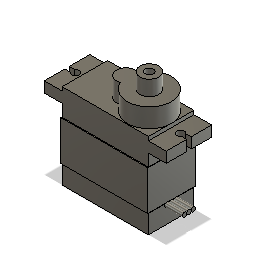
MG90_Rebuild (Autodesk Fusion 360 design; units mm, degrees)
Autodesk Fusion 360 part; units mm, degrees
note: some values were not read from the file. Set by a fixed rule: which sketch regions a step uses.
sketch "ServoRotatingPlate" plane through (0, 0, 0) normal (0, 1, 0) x (1, 0, 0)
  circle A0 centre (0, 0) radius 5.8
  line L0 (5.75, 6) -> (-17.05, 6)
  line L1 (-17.05, 6) -> (-17.05, -6)
  line L2 (-17.05, -6) -> (5.75, -6)
  line L3 (5.75, -6) -> (5.75, 6)
  line L4 (-8.7, 0) -> (5.75, 0) construction
  circle A1 centre (-6.2, 0) radius 2.5
  circle A2 centre (0, 0) radius 2.5
  circle A3 centre (0, 0) radius 1.1
  point P0 (5.8, 0)
  dimension "d4" = 11.6
  dimension "d6" = 12
  dimension "d7" = 22.8
  dimension "d10" = 5
  dimension "d12" = 14.5
  dimension "d13" = 5.75
  dimension "d14" = 8.1
  dimension "d48" = 5
  dimension "d49" = 1.4
  constraint coincident A0.centre A2.centre
  constraint horizontal L0
  constraint vertical L1
  constraint horizontal L2
  constraint vertical L3
  constraint horizontal L4
  constraint midpoint L3 L4.end
  constraint coincident L4 A1.centre
  constraint coincident L4.start A1
  constraint coincident A0.centre L4
  constraint coincident L4 P0
  constraint coincident A0 P0
  constraint concentric A0 A2
  constraint concentric A2 A3
  measures "d4" diameter of A0
  measures "d6" distance of L0.start L2.end
  measures "d7" distance of L0.start L0.end
  measures "d10" diameter of A1
  measures "d12" distance of L4.start P0
  measures "d13" distance of A0.centre L3
  measures "d48" diameter of A2
  measures "d49" distance of A2 A3
extrude "Extrude1" add sketch "ServoRotatingPlate" against normal blind 5 contours A0 L3 | A0 L3 A1 | A0 A1 | A0 A1 | A2 | A3
extrude "Extrude2" add sketch "ServoRotatingPlate" against normal blind 22.5 from surface at -5 contours A0 L3 A1 | A0 L0 L1 L2 L3 A1 | A0 A1 | A0 A1 | A2 | A3
ref_plane "WorkPlane1" through (-5.65, -6, 0) normal (0, 1, 0) x (0, 0, 1)
sketch "EarBase" plane through (-5.65, -6, 0) normal (0, 1, 0) x (1, 0, 0)
  line L0 (16.1, 6) -> (-16.1, 6)
  line L1 (-16.1, 6) -> (-16.1, -6)
  line L2 (-16.1, -6) -> (16.1, -6)
  line L3 (16.1, -6) -> (16.1, 6)
  line L4 (16.1, 6) -> (-16.1, -6) construction
  line L5 (-16.1, 6) -> (16.1, -6) construction
  line L6 (-16.1, 0) -> (16.1, 0) construction
  circle A0 centre (-13.9, 0) radius 1
  line L7 (-14.7, 0.6) -> (-16.1, 0.6)
  line L8 (-14.7, -0.6) -> (-16.1, -0.6)
  line L9 (-11.4, 6) -> (-11.4, -6)
  line L10 (0, 0) -> (0, 6) construction
  line L11 (14.7, 0.6) -> (16.1, 0.6)
  circle A1 centre (13.9, 0) radius 1
  line L12 (14.7, -0.6) -> (16.1, -0.6)
  point P0 (11.4, 6)
  dimension "d26" = 32.2
  dimension "d31" = 2
  dimension "d33" = 1.2
  dimension "d34" = 2.5
  dimension "d35" = 4.7
  constraint perpendicular L0 L1
  constraint parallel L0 L2
  constraint parallel L1 L3
  constraint horizontal L0
  constraint coincident L4 L10.start
  constraint coincident L5 L10.start
  constraint coincident L10.start origin
  constraint coincident L0 P0
  constraint midpoint L1 L6.start
  constraint midpoint L3 L6.end
  constraint coincident L6 A0.centre
  constraint coincident A0 L7.start
  constraint coincident L1 L7.end
  constraint perpendicular L1 L7
  constraint symmetric L6 L7.start L8.start
  constraint symmetric L6 L7.end L8.end
  constraint midpoint L0 L10.end
  constraint symmetric A0 L10 A1
  constraint symmetric L7.start L10 L11.start
  constraint symmetric L7.end L10 L11.end
  constraint symmetric L8.start L10 L12.start
  constraint symmetric L8.end L10 L12.end
  measures "d26" distance of L0.start L0.end
  measures "d31" diameter of A0
  measures "d33" distance of L7.end L8.end
  measures "d34" distance of A0.centre L9
  measures "d35" distance of L0.end L9.start
extrude "Extrude3" add sketch "EarBase" against normal blind 2.8 contours L0 L2 L3 L9 L11 A1 L12 | L0 L1 L2 A0 L7 L8 L9
ref_plane "WorkPlane2" through (-5.65, -22.5, 0) normal (0, -1, 0) x (0, 0, -1)
sketch "StickerBase" plane through (-5.65, -22.5, 0) normal (0, -1, 0) x (1, 0, 0)
  line L0 (11.5, -6.25) -> (-11.5, -6.25)
  line L1 (-11.5, -6.25) -> (-11.5, 6.25)
  line L2 (-11.5, 6.25) -> (11.5, 6.25)
  line L3 (11.5, 6.25) -> (11.5, -6.25)
  line L4 (11.5, -6.25) -> (-11.5, 6.25) construction
  line L5 (-11.5, -6.25) -> (11.5, 6.25) construction
  dimension "d42" = 23
  dimension "d43" = 12.5
  constraint perpendicular L0 L1
  constraint parallel L0 L2
  constraint parallel L1 L3
  constraint horizontal L0
  constraint coincident L4 origin
  constraint coincident L5 origin
  measures "d42" distance of L0.start L0.end
  measures "d43" distance of L0.start L2.end
extrude "Extrude4" add sketch "StickerBase" against normal blind 10.5
extrude "Extrude5" add sketch "ServoRotatingPlate" along normal blind 4 contours A2
sketch "WireHardCoded" plane through (5.75, 0, 0) normal (1, 0, 0) x (0, 0, -1)
  line L0 (6, -22.5) -> (-6, -22.5)
  line L1 (-6, -22.5) -> (-6, -27.5)
  line L2 (-6, -27.5) -> (6, -27.5)
  line L3 (6, -27.5) -> (6, -22.5)
  line L4 (-1.75, -23.5) -> (1.75, -23.5) construction
  line L5 (1.75, -23.5) -> (1.75, -22.3333) construction
  line L6 (1.75, -22.3333) -> (-1.75, -22.3333) construction
  line L7 (-1.75, -22.3333) -> (-1.75, -23.5) construction
  line L8 (0, -27.5) -> (0, -23.5) construction
  line L9 (-1.75, -22.9167) -> (1.75, -22.9167) construction
  circle A0 centre (0, -22.9167) radius 0.5833
  circle A1 centre (-1.17, -22.9167) radius 0.5833
  circle A2 centre (1.17, -22.9167) radius 0.5833
  dimension "d52" = 1.1667
  dimension "d53" = 3.5
  dimension "d54" = 4
  dimension "d57" = 1.17
  dimension "d58" = 0
  constraint horizontal L4
  constraint vertical L5
  constraint horizontal L6
  constraint vertical L7
  constraint midpoint L2 L8.start
  constraint midpoint L4 L8.end
  constraint vertical L8
  constraint midpoint L7 L9.start
  constraint midpoint L5 L9.end
  constraint midpoint L9 A0.centre
  constraint tangent L6 A0
  measures "d52" distance of L4.end L5.end
  measures "d53" distance of L4.start L4.end
  measures "d54" distance of L8.start L8.end
extrude "Extrude6" add sketch "WireHardCoded" along normal up to surface (4.7 mm away) contours L0 A2 | L0 A2 | L0 A0 | L0 A0 | L0 A1 | L0 A1
equation "Note0 = 0" comment "The [0,0,0] is placed at the servo shaft base plane, for better alignment"
equation "Note1 = 1" comment "Improvement for https://www.thingiverse.com/thing:2641076"
equation "BaseCircleD = 11.6 mm"
equation "d4 = BaseCircleD"
equation "BaseRectW = 12 mm"
equation "d6 = BaseRectW"
equation "d7 = BaseRectH"
equation "BaseRectH = 22.8 mm"
equation "BaseCircle2D = 5 mm"
equation "d10 = BaseCircle2D"
equation "E2EDist = 14.5 mm"
equation "d12 = E2EDist"
equation "d13 = CenterMeasureL"
equation "CenterMeasureL = 5.75 mm"
equation "GearIsleHeight = 5 mm"
equation "d17 = -GearIsleHeight"
equation "BoxHeight = 22.5 mm"
equation "d21 = -BoxHeight"
equation "Ear_Down = 1 mm"
equation "d24 = -Ear_Down"
equation "Ear_L = 32.2 mm"
equation "d26 = Ear_L"
equation "Ear_Thick = 2.8 mm"
equation "d28 = -Ear_Thick"
equation "EarScrew_D = 2 mm"
equation "d31 = EarScrew_D"
equation "Ear_Slit = 1.2 mm"
equation "d33 = Ear_Slit"
equation "d34 = HolePos"
equation "HolePos = 2.5 mm"
equation "sticker_height = 10.5 mm"
equation "stick_pos = 5 mm"
equation "d39 = -stick_pos"
equation "Sticker_Profile_L = 23 mm"
equation "Sticker_Profile_W = 12.5 mm"
equation "d42 = Sticker_Profile_L"
equation "d43 = Sticker_Profile_W"
equation "d44 = -sticker_height"
equation "ServoShaftProf = 5 mm"
equation "ServoProfHeight = 4 mm"
equation "d48 = ServoShaftProf"
equation "d50 = ServoProfHeight"
equation "d52 = ( 3.5 / 3 ) * 1 mm"
named bodies: "WireHardCoded"
